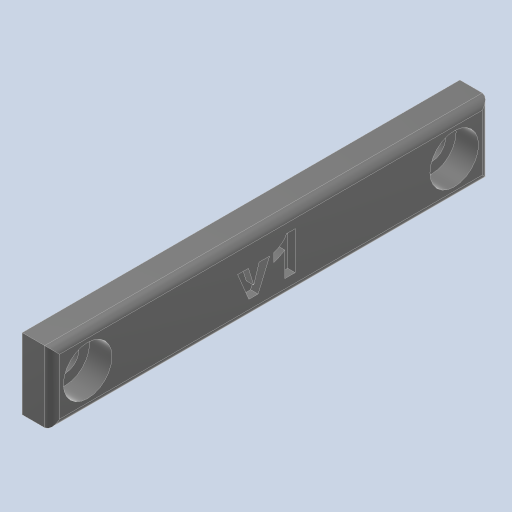
# Autodesk Inventor part: wb_holder_inside_01
Saved by Autodesk Inventor 2024.4 (Build 284460000, 460)
## iProperties
Created: 2026-05-05
Part Number: wb_holder_inside_01
Material: PLA Black
Document SubType Name: Modeling
Designer: tooles01
Density: 1.06 g/cm^3
Appearance: Smooth - White(2)
Author: tooles01
Autodesk Inventor part; units mm, degrees
ref_plane "YZ Plane" through (0, 0, 0) normal (1, 0, 0) x (0, 1, 0)
ref_plane "XZ Plane" through (0, 0, 0) normal (0, 1, 0) x (-1, 0, 0)
ref_plane "XY Plane" through (0, 0, 0) normal (0, 0, 1) x (1, 0, 0)
derived "wb_holder_outside_01.ipt"
sketch "Sketch1" plane through (0, 0, 0) normal (1, 0, 0) x (0, 1, 0)
  line L0 (7.6312, 29.25) -> (-1.8688, 29.25)
  line L1 (-1.8688, 29.25) -> (-1.8688, -29.25)
  line L2 (-1.8688, -29.25) -> (7.6312, -29.25)
  line L3 (7.6312, -29.25) -> (7.6312, 29.25)
  circle A0 centre (2.8812, -24.5) radius 1.85
  circle A1 centre (2.8812, 24.5) radius 1.85
  ellipse E0 centre (2.8812, 24.5) end of major axis (2.8812, 26.6) minor radius 2.0376 construction
  ellipse E1 centre (2.8812, -24.5) end of major axis (2.8812, -22.4) minor radius 2.0376 construction
  point P0 (0, 0)
  point P1 (2.8812, 29.25)
  dimension "d1" = 3.7
  dimension "d2" = 4.75
  dimension "d3" = 4.75
  dimension "d4" = 4.75
  constraints: 8 end point, 3 perpendicular, 2 centre point, 2 coincident, 1 equal radius, 1 midpoint, 1 vertical, 1 vertical alignment
  measures "d1" diameter of A1
  measures "d2" distance from line of L0 A1.centre
  measures "d3" distance from line of L2 A0.centre
  measures "d4" distance from line of L3 A1.centre
sketch "Sketch3: heat-set inserts" plane through (-29, -1, -30) normal (-0.9702957, -0.2419219, 0) x (0, 0, 1)
  circle A0 centre (5.5, 4) radius 2.1
  circle A1 centre (54.5, 4) radius 2.1
  line L0 (30, 0) -> (30, 8) construction
  line L1 (0, 0) -> (0, 8) construction
  line L2 (60, 8) -> (60, 0) construction
  line L3 (0, 8) -> (60, 8) construction
  line L4 (60, 0) -> (0, 0) construction
  point P0 (30, -6.0454)
  point P1 (0, 4)
sketch "Sketch3: text" plane through (0, 0, 0) normal (1, 0, 0) x (0, 1, 0)
  line L0 (4.8812, 2) -> (4.8812, -2) construction
  line L1 (4.8812, -2) -> (0.8812, -2) construction
  line L2 (0.8812, -2) -> (0.8812, 2) construction
  line L3 (0.8812, 2) -> (4.8812, 2) construction
  line L4 (7.6312, -29.25) -> (7.6312, 29.25) construction
  line L5 (7.6312, 29.25) -> (-1.8688, 29.25) construction
  line L6 (3.9615, 4.4562) -> (3.9615, 3.0125)
  line L7 (3.9615, 3.0125) -> (1.6661, 2.3051)
  line L8 (1.6661, 2.3051) -> (3.9615, 1.5784)
  line L9 (3.9615, 1.5784) -> (3.9615, 0.1781)
  line L10 (3.9615, 0.1781) -> (0.3379, 1.718)
  line L11 (0.3379, 1.718) -> (0.3379, 2.95)
  line L12 (0.3379, 2.95) -> (3.9615, 4.4562)
  line L13 (5.4245, -3.2387) -> (0.3379, -3.2387)
  line L14 (0.3379, -3.2387) -> (0.3379, -1.8335)
  line L15 (0.3379, -1.8335) -> (3.6728, -1.8335)
  spline S0 degree 2 poles (3.6728, -1.8335) (3.4129, -1.4918) (3.0953, -0.8566) (2.9461, -0.3754) knots 0 0 0 1 2 2 2
  line L16 (2.9461, -0.3754) -> (4.0867, -0.3754)
  spline S1 degree 2 poles (4.0867, -0.3754) (4.3128, -1.0828) (4.9529, -1.8672) (5.4245, -2.0885) knots 0 0 0 1 2 2 2
  line L17 (5.4245, -2.0885) -> (5.4245, -3.2387)
  point P0 (0, 0)
  point P1 (4.8812, 0)
  point P2 (7.6312, 0)
  point P3 (2.8812, 2)
  point P4 (2.8812, 29.25)
  dimension "d15" = 4
  constraints: 4 midpoint, 1 horizontal, 1 horizontal alignment, 1 perpendicular, 1 vertical alignment, 2 other
  measures "d15" distance of L2.end L0.start
extrude "Ex1: base" add sketch "Sketch1" against normal blind 4 contours L3 L2 L1 L0 | A0 | A1
hole "Hole1" at (0, 2.8812, -24.5) at (0, 2.8812, 24.5) direction (-1, 0, 0) diameter 3.7 end through all counterbore diameter 6.5 counterbore depth 3 clearance for "Socket Head Cap Screw" size "M3" standard "Ansi Metric M Profile"
fillet "Fillet1" radius 1 4 edges at (0, 7.6312, 0) (0, 2.8812, 29.25) (0, -1.8688, 0) (0, 2.8812, -29.25)
extrude "Extrusion2" cut sketch "Sketch3: text" against normal blind 1
equation "\"d3\" = d2"
equation "\"d4\" = d2"
body "Solid1"
